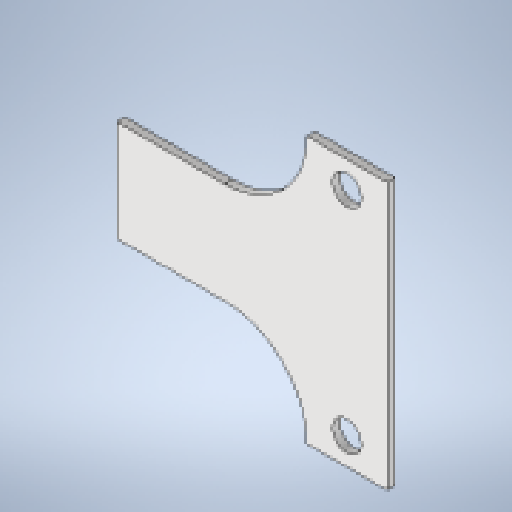
# Autodesk Inventor part: MSC 815 wall inner
Saved by Autodesk Inventor 2025 (Build 290162010, 162A)
## iProperties
Created: 2024-04-18
Part Number: MSC 815 wall inner
Material: AISI304
Document SubType Name: Sheet Metal
Designer: admin
Stock Number: МОО 813 стойка боковая жабры
Mass: 2919.69 g
Surface Area: 2571.84 cm^2
Volume: 364.962 cm^3
Density: 8 g/cm^3
Flat Pattern Width: 9 cm
Flat Pattern Length: 11 cm
Flat Pattern Area: 99 cm^2
Sheet Metal Rule: AISI304 3mm
Sheet Metal Width: 90,000 mm
Sheet Metal Length: 110,000 mm
Sheet Metal Area: 9900,000 mm^2
Appearance: Default
Author: admin
Autodesk Inventor part; units mm, degrees
ref_plane "YZ Plane" through (0, 0, 0) normal (1, 0, 0) x (0, 1, 0)
ref_plane "XZ Plane" through (0, 0, 0) normal (0, 1, 0) x (-1, 0, 0)
ref_plane "XY Plane" through (0, 0, 0) normal (0, 0, 1) x (1, 0, 0)
sketch "Sketch1" plane through (0, 0, 0) normal (0, 0, 1) x (1, 0, 0)
  line L0 (-15, 55) -> (15, 55)
  line L1 (15, 55) -> (15, -55)
  line L2 (15, -55) -> (-15, -55)
  line L3 (-15, -55) -> (-15, 55)
  line L4 (-15, 55) -> (15, -55) construction
  line L5 (15, 55) -> (-15, -55) construction
  line L6 (-15, 19) -> (-75, 19)
  line L7 (-75, 19) -> (-75, -19)
  line L8 (-75, -19) -> (-15, -19)
  line L9 (-15, -19) -> (-15, 19)
  arc A0 (-51, 19) -> (-15, 55) centre (-51, 55) ccw
  arc A1 (-15, -55) -> (-51, -19) centre (-51, -55) ccw
  circle A2 centre (0, 40) radius 5.5
  circle A3 centre (0, -40) radius 5.5
  line L10 (0, 0) -> (15, 0) construction
  point P0 (-75, 0)
  dimension "d157" = 30
  dimension "d158" = 110
  dimension "d159" = 38
  dimension "d160" = 80
  dimension "d161" = 11
  dimension "d162" = 60
  measures "d157" distance of L0.start L0.end
  measures "d158" distance of L0.end L1.end
  measures "d159" distance of L6.end L7.end
  measures "d160" distance of A3.centre A2.centre
  measures "d161" diameter of A2
  measures "d162" distance between parallel lines of L3 L7
extrude "Plate3" add sketch "Sketch1" along normal blind 3
fillet "Corner Round2" radius 6 4 edges at (-15, 55, 1.5) (15, 55, 1.5) (-15, -55, 1.5) (15, -55, 1.5)
equation "\"BendReliefWidth\" = Thickness"
equation "\"BendReliefDepth\" = 0.5 * Thickness"
equation "\"CornerReliefSize\" = 4 * Thickness"
equation "\"MinimumRemnant\" = 2 * Thickness"
equation "\"GapSize\" = Thickness"
equation "\"Thickness\" = 3"
body "Solid4"
